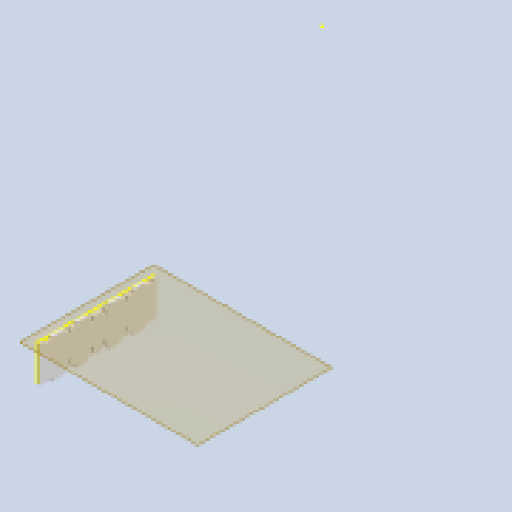
# Autodesk Inventor part: стенка
Saved by Autodesk Inventor 2024.2 (Build 282272000, 272)
## iProperties
Created: 2025-12-09
Part Number: стенка
Material: Типовые
Document SubType Name: Modeling
Designer: katya_notebook
Mass: 65.1748 g
Surface Area: 247.334 cm^2
Volume: 65.1748 cm^3
Density: 1 g/cm^3
Appearance: По умолчанию
Author: katya_notebook
Autodesk Inventor part; units mm, degrees
ref_plane "YZ Plane" through (0, 0, 0) normal (1, 0, 0) x (0, 1, 0)
ref_plane "XZ Plane" through (0, 0, 0) normal (0, 1, 0) x (-1, 0, 0)
ref_plane "РабПлоскость1" through (-475.2675, -216.9886, 379.0883) normal (0, 1, 0) x (-1, 0, 0)
sketch "Эскиз1" plane through (-475.2675, -216.9886, 379.0883) normal (0, 1, 0) x (-1, 0, 0)
  line L0 (135, 97.5) -> (129, 97.5)
  line L1 (129, 97.5) -> (129, -97.5)
  line L2 (129, -97.5) -> (135, -97.5)
  line L3 (135, -97.5) -> (135, 97.5)
  line L4 (135, -97.5) -> (135, 97.5) projected
  line L5 (127, 97.5) -> (62.5237, 97.5) projected
  line L6 (62.5237, -97.5) -> (127, -97.5) projected
  point P0 (-475.2675, -379.0883)
  dimension "d0" = 0
  dimension "d1" = 6
  dimension "d2" = 0
  dimension "d3" = 0
  constraints: 8 end point, 2 parallel, 1 horizontal, 1 perpendicular, 1 vertical alignment
  measures "d0" horizontal extent of L3
  measures "d1" distance of L0.start L0.end
  measures "d2" distance between parallel lines of L6 L2
  measures "d3" distance between parallel lines of L0 L5
ref_plane "РабПлоскость2" through (-610.2675, -276.6936, 277.5883) normal (0, 1, 0) x (0, 0, 1)
extrude "Выдавливание1" add sketch "Эскиз1" against normal up to surface (59.705 mm away)
sketch "Эскиз2" plane through (-610.2675, -216.9886, 281.5883) normal (-1, 0, 0) x (0, 0, 1)
  line L0 (175, -4) -> (187, -4) projected
  line L1 (195, 0) -> (195, -59.705) projected
  line L2 (0, 0) -> (195, 0) projected
  line L3 (0, 0) -> (0, -59.705) projected
  point P0 (-281.5883, 216.9886)
  point P1 (195, -59.705)
  point P2 (0, -59.705)
  constraints: 2 other
sketch "Эскиз3" plane through (-610.2675, -276.6936, 281.5883) normal (-1, 0, 0) x (0, 0, 1)
  line L0 (195, 0) -> (0, 0) projected
  line L1 (175, 0) -> (155, 0)
  line L2 (155, 0) -> (155, -5)
  line L3 (155, -5) -> (175, -5)
  line L4 (175, -5) -> (175, 0)
  line L5 (195, 59.705) -> (195, 0) projected
  line L6 (135, 0) -> (115, 0)
  line L7 (115, 0) -> (115, -5)
  line L8 (115, -5) -> (135, -5)
  line L9 (135, -5) -> (135, 0)
  line L10 (20, 0) -> (40, 0)
  line L11 (40, 0) -> (40, -5)
  line L12 (40, -5) -> (20, -5)
  line L13 (20, -5) -> (20, 0)
  line L14 (60, 0) -> (80, 0)
  line L15 (80, 0) -> (80, -5)
  line L16 (80, -5) -> (60, -5)
  line L17 (60, -5) -> (60, 0)
  line L18 (97.5, 27.8525) -> (226.4185, 27.8525)
  line L19 (195, 55.705) -> (0, 55.705)
  line L20 (175, 55.705) -> (155, 55.705)
  line L21 (155, 55.705) -> (155, 60.705)
  line L22 (155, 60.705) -> (175, 60.705)
  line L23 (175, 60.705) -> (175, 55.705)
  line L24 (135, 55.705) -> (115, 55.705)
  line L25 (115, 55.705) -> (115, 60.705)
  line L26 (115, 60.705) -> (135, 60.705)
  line L27 (135, 60.705) -> (135, 55.705)
  line L28 (20, 55.705) -> (40, 55.705)
  line L29 (40, 55.705) -> (40, 60.705)
  line L30 (40, 60.705) -> (20, 60.705)
  line L31 (20, 60.705) -> (20, 55.705)
  line L32 (60, 55.705) -> (80, 55.705)
  line L33 (80, 55.705) -> (80, 60.705)
  line L34 (80, 60.705) -> (60, 60.705)
  line L35 (60, 60.705) -> (60, 55.705)
  point P0 (-281.5883, 276.6936)
  point P1 (40, 55.705)
  point P2 (80, 55.705)
  point P3 (40, 0)
  point P4 (80, 0)
  point P5 (115, 55.705)
  point P6 (155, 55.705)
  point P7 (115, 0)
  point P8 (155, 0)
  dimension "d8" = 5
  dimension "d9" = 20
  dimension "d10" = 20
  dimension "d11" = 20
  dimension "d12" = 20
  dimension "d13" = 5
  dimension "d14" = 20
  dimension "d15" = 20
  dimension "d16" = 20
  dimension "d17" = 20
  dimension "d43" = 5
  constraints: 68 end point, 17 symmetric about line, 8 parallel, 8 point on line, 5 horizontal, 4 perpendicular
  measures "d8" distance of L3.end L1.start
  measures "d9" distance of L2.end L3.end
  measures "d10" distance of L0.start L1.start
  measures "d11" distance of L7.end L8.end
  measures "d12" distance of L1.end L6.start
  measures "d13" distance of L10.end L11.end
  measures "d14" distance of L11.end L12.end
  measures "d15" distance of L10.start L0.end
  measures "d16" distance of L15.end L16.end
  measures "d17" distance of L14.start L10.end
  measures "d43" distance of L16.end L14.start
extrude "Выдавливание3" add sketch "Эскиз3" against normal blind 6
sketch "Эскиз4" plane through (-610.2675, -276.6936, 281.5883) normal (-1, 0, 0) x (0, 0, 1)
  point P0 (-281.5883, 276.6936)
sketch "Эскиз5" plane through (-610.2675, -276.6936, 281.5883) normal (-1, 0, 0) x (0, 0, 1)
  point P0 (-281.5883, 276.6936)
sketch "Эскиз6" plane through (-610.2675, -276.6936, 281.5883) normal (-1, 0, 0) x (0, 0, 1)
  line L0 (111.125, 1.5) -> (104.625, 1.5)
  line L1 (104.625, 1.5) -> (104.625, 4.5)
  line L2 (104.625, 4.5) -> (111.125, 4.5)
  line L3 (111.125, 4.5) -> (111.125, 1.5)
  line L4 (115, 0) -> (115, -5) projected
  line L5 (90.375, 1.5) -> (83.875, 1.5)
  line L6 (83.875, 1.5) -> (83.875, 4.5)
  line L7 (83.875, 4.5) -> (90.375, 4.5)
  line L8 (90.375, 4.5) -> (90.375, 1.5)
  line L9 (111.125, 3) -> (104.625, 3)
  line L10 (115, 0) -> (80, 0) projected
  line L11 (106.125, 6) -> (109.625, 6)
  line L12 (109.625, 6) -> (109.625, 0)
  line L13 (109.625, 0) -> (106.125, 0)
  line L14 (106.125, 0) -> (106.125, 6)
  line L15 (106.125, 6) -> (109.625, 0) construction
  line L16 (109.625, 6) -> (106.125, 0) construction
  line L17 (90.375, 3) -> (83.875, 3)
  line L18 (87.125, 1.5) -> (87.125, 4.5)
  line L19 (85.375, 6) -> (88.875, 6)
  line L20 (88.875, 6) -> (88.875, 0)
  line L21 (88.875, 0) -> (85.375, 0)
  line L22 (85.375, 0) -> (85.375, 6)
  line L23 (85.375, 6) -> (88.875, 0) construction
  line L24 (88.875, 6) -> (85.375, 0) construction
  line L25 (148.25, 1.5) -> (141.75, 1.5)
  line L26 (141.75, 1.5) -> (141.75, 4.5)
  line L27 (141.75, 4.5) -> (148.25, 4.5)
  line L28 (148.25, 4.5) -> (148.25, 1.5)
  line L29 (148.25, 3) -> (141.75, 3)
  line L30 (143.25, 12) -> (146.75, 12)
  line L31 (146.75, 12) -> (146.75, -6)
  line L32 (146.75, -6) -> (143.25, -6)
  line L33 (143.25, -6) -> (143.25, 12)
  line L34 (143.25, 12) -> (146.75, -6) construction
  line L35 (146.75, 12) -> (143.25, -6) construction
  line L36 (155, 0) -> (155, -5) projected
  line L37 (53.25, 1.5) -> (46.75, 1.5)
  line L38 (46.75, 1.5) -> (46.75, 4.5)
  line L39 (46.75, 4.5) -> (53.25, 4.5)
  line L40 (53.25, 4.5) -> (53.25, 1.5)
  line L41 (53.25, 3) -> (46.75, 3)
  line L42 (48.25, 12) -> (51.75, 12)
  line L43 (51.75, 12) -> (51.75, -6)
  line L44 (51.75, -6) -> (48.25, -6)
  line L45 (48.25, -6) -> (48.25, 12)
  line L46 (48.25, 12) -> (51.75, -6) construction
  line L47 (51.75, 12) -> (48.25, -6) construction
  line L48 (60, 0) -> (60, -5) projected
  line L49 (195, 59.705) -> (195, 0) projected
  line L50 (195, 29.8525) -> (88.875, 29.8525)
  line L51 (111.125, 58.205) -> (104.625, 58.205)
  line L52 (104.625, 58.205) -> (104.625, 55.205)
  line L53 (104.625, 55.205) -> (111.125, 55.205)
  line L54 (111.125, 55.205) -> (111.125, 58.205)
  line L55 (115, 59.705) -> (115, 64.705)
  line L56 (90.375, 58.205) -> (83.875, 58.205)
  line L57 (83.875, 58.205) -> (83.875, 55.205)
  line L58 (83.875, 55.205) -> (90.375, 55.205)
  line L59 (90.375, 55.205) -> (90.375, 58.205)
  line L60 (111.125, 56.705) -> (104.625, 56.705)
  line L61 (115, 59.705) -> (80, 59.705)
  line L62 (106.125, 53.705) -> (109.625, 53.705)
  line L63 (109.625, 53.705) -> (109.625, 59.705)
  line L64 (109.625, 59.705) -> (106.125, 59.705)
  line L65 (106.125, 59.705) -> (106.125, 53.705)
  line L66 (106.125, 53.705) -> (109.625, 59.705) construction
  line L67 (109.625, 53.705) -> (106.125, 59.705) construction
  line L68 (90.375, 56.705) -> (83.875, 56.705)
  line L69 (87.125, 58.205) -> (87.125, 55.205)
  line L70 (85.375, 53.705) -> (88.875, 53.705)
  line L71 (88.875, 53.705) -> (88.875, 59.705)
  line L72 (88.875, 59.705) -> (85.375, 59.705)
  line L73 (85.375, 59.705) -> (85.375, 53.705)
  line L74 (85.375, 53.705) -> (88.875, 59.705) construction
  line L75 (88.875, 53.705) -> (85.375, 59.705) construction
  line L76 (146.75, 65.705) -> (143.25, 65.705)
  line L77 (146.75, 47.705) -> (146.75, 65.705)
  line L78 (146.75, 47.705) -> (143.25, 65.705) construction
  line L79 (143.25, 47.705) -> (146.75, 65.705) construction
  line L80 (143.25, 65.705) -> (143.25, 47.705)
  line L81 (141.75, 58.205) -> (141.75, 55.205)
  line L82 (148.25, 58.205) -> (141.75, 58.205)
  line L83 (148.25, 55.205) -> (148.25, 58.205)
  line L84 (141.75, 55.205) -> (148.25, 55.205)
  line L85 (148.25, 56.705) -> (141.75, 56.705)
  line L86 (143.25, 47.705) -> (146.75, 47.705)
  line L87 (155, 59.705) -> (155, 64.705)
  line L88 (51.75, 65.705) -> (48.25, 65.705)
  line L89 (51.75, 47.705) -> (51.75, 65.705)
  line L90 (51.75, 47.705) -> (48.25, 65.705) construction
  line L91 (48.25, 47.705) -> (51.75, 65.705) construction
  line L92 (48.25, 65.705) -> (48.25, 47.705)
  line L93 (46.75, 58.205) -> (46.75, 55.205)
  line L94 (53.25, 58.205) -> (46.75, 58.205)
  line L95 (53.25, 55.205) -> (53.25, 58.205)
  line L96 (46.75, 55.205) -> (53.25, 55.205)
  line L97 (53.25, 56.705) -> (46.75, 56.705)
  line L98 (48.25, 47.705) -> (51.75, 47.705)
  line L99 (60, 59.705) -> (60, 64.705)
  line L100 (109.625, 6) -> (106.125, 6)
  line L101 (106.125, 6) -> (106.125, 12)
  line L102 (106.125, 12) -> (109.625, 12)
  line L103 (109.625, 12) -> (109.625, 6)
  line L104 (88.875, 6) -> (85.375, 6)
  line L105 (85.375, 6) -> (85.375, 12)
  line L106 (85.375, 12) -> (88.875, 12)
  line L107 (88.875, 12) -> (88.875, 6)
  line L108 (109.625, 53.705) -> (106.125, 53.705)
  line L109 (106.125, 53.705) -> (106.125, 47.705)
  line L110 (106.125, 47.705) -> (109.625, 47.705)
  line L111 (109.625, 47.705) -> (109.625, 53.705)
  line L112 (88.875, 53.705) -> (85.375, 53.705)
  line L113 (85.375, 53.705) -> (85.375, 47.705)
  line L114 (85.375, 47.705) -> (88.875, 47.705)
  line L115 (88.875, 47.705) -> (88.875, 53.705)
  point P0 (-281.5883, 276.6936)
  point P1 (115, -2.5)
  point P2 (107.875, 11.6549)
  point P3 (107.875, 3)
  point P4 (99.25, 0)
  point P5 (87.125, 3)
  point P6 (149.0518, 14.6563)
  point P7 (145, 3)
  point P8 (155, -2.5)
  point P9 (49.2049, 25.9501)
  point P10 (50, 3)
  point P11 (60, -2.5)
  point P12 (48.25, 4.5)
  point P13 (48.25, 1.5)
  point P14 (51.75, 1.5)
  point P15 (51.75, 4.5)
  point P16 (88.875, 4.5)
  point P17 (85.375, 4.5)
  point P18 (85.375, 1.5)
  point P19 (85.375, 0)
  point P20 (88.875, 1.5)
  point P21 (106.125, 1.5)
  point P22 (106.125, 0)
  point P23 (109.625, 1.5)
  point P24 (109.625, 4.5)
  point P25 (106.125, 4.5)
  point P26 (143.25, 1.5)
  point P27 (146.75, 1.5)
  point P28 (146.75, 4.5)
  point P29 (143.25, 4.5)
  point P30 (195, 55.705)
  point P31 (115, 62.205)
  point P32 (107.875, 48.0501)
  point P33 (107.875, 56.705)
  point P34 (99.25, 59.705)
  point P35 (87.125, 56.705)
  point P36 (145, 56.705)
  point P37 (149.0518, 45.0486)
  point P38 (155, 62.205)
  point P39 (50, 56.705)
  point P40 (60, 62.205)
  point P41 (51.75, 55.205)
  point P42 (51.75, 58.205)
  point P43 (48.25, 58.205)
  point P44 (48.25, 55.205)
  point P45 (88.875, 55.205)
  point P46 (88.875, 58.205)
  point P47 (85.375, 55.705)
  point P48 (85.375, 58.205)
  point P49 (85.375, 55.205)
  point P50 (106.125, 58.205)
  point P51 (106.125, 55.205)
  point P52 (109.625, 55.205)
  point P53 (109.625, 58.205)
  point P54 (143.25, 58.205)
  point P55 (143.25, 55.205)
  point P56 (146.75, 55.205)
  point P57 (146.75, 58.205)
  point P58 (85.375, 59.705)
  point P59 (85.375, 53.705)
  point P60 (106.125, 53.705)
  point P61 (85.375, 6)
  point P62 (106.125, 6)
  point P63 (85.375, 0)
  point P64 (85.375, 59.705)
  point P65 (85.375, 53.705)
  point P66 (85.375, 6)
  dimension "d0" = 0
  dimension "d20" = 6.5
  dimension "d21" = 3
  dimension "d22" = 3.875
  dimension "d26" = 6.5
  dimension "d27" = 3
  dimension "d29" = 3
  dimension "d30" = 3.5
  dimension "d32" = 3.5
  dimension "d33" = 6.5
  dimension "d34" = 3
  dimension "d35" = 3.5
  dimension "d36" = 8.25
  dimension "d37" = 6.5
  dimension "d38" = 3
  dimension "d39" = 3.5
  dimension "d40" = 8.25
  dimension "d46" = 6
  dimension "d47" = 6
  constraints: 222 end point, 59 symmetric about line, 26 midpoint, 24 parallel, 13 horizontal, 13 perpendicular, 6 point on line, 5 collinear
  measures "d20" distance of L0.start L0.end
  measures "d21" distance of L0.end L1.end
  measures "d22" horizontal distance of L9.start point (115, -2.5)
  measures "d26" distance of L5.start L5.end
  measures "d27" distance of L5.end L6.end
  measures "d29" distance from line of L10 point (107.875, 3)
  measures "d30" distance of L12.end L13.end
  measures "d32" distance of L21.end L20.end
  measures "d33" distance of L25.start L26.start
  measures "d34" distance of L26.start L26.end
  measures "d35" distance of L32.start L32.end
  measures "d36" distance from line of L31 point (155, -2.5)
  measures "d37" distance of L37.start L38.start
  measures "d38" distance of L38.start L38.end
  measures "d39" distance of L44.start L44.end
  measures "d40" distance from line of L43 point (60, -2.5)
  measures "d46" distance of L100.end L101.end
  measures "d47" distance of L108.end L109.end
extrude "Выдавливание4" cut sketch "Эскиз6" against normal blind 6
sketch "Эскиз7" plane through (-610.2675, -276.6936, 281.5883) normal (-1, 0, 0) x (0, 0, 1)
  line L0 (175, 55.705) -> (187, 55.705) projected
  line L1 (195, 59.705) -> (195, 0) projected
  line L2 (175, 59.705) -> (195, 59.705) projected
  line L3 (175, 59.705) -> (175, 55.705) projected
  line L4 (155, 55.705) -> (155, 59.705) projected
  line L5 (135, 55.705) -> (155, 55.705) projected
  line L6 (135, 59.705) -> (135, 55.705) projected
  line L7 (135, 59.705) -> (155, 59.705) projected
  line L8 (80, 55.705) -> (115, 55.705) projected
  line L9 (115, 55.705) -> (115, 59.705) projected
  line L10 (80, 59.705) -> (80, 55.705) projected
  line L11 (80, 59.705) -> (115, 59.705) projected
  line L12 (60, 55.705) -> (60, 59.705) projected
  line L13 (40, 55.705) -> (60, 55.705) projected
  line L14 (40, 59.705) -> (60, 59.705) projected
  line L15 (40, 59.705) -> (40, 55.705) projected
  line L16 (175, 55.705) -> (187, 55.705) projected
  line L17 (0, 59.705) -> (20, 59.705) projected
  line L18 (0, 59.705) -> (0, 0) projected
  point P0 (-281.5883, 276.6936)
  point P1 (195, 0)
  point P2 (0, 0)
  point P3 (175, 59.705)
  constraints: 2 other
extrude "Выдавливание5" cut sketch "Эскиз7" against normal blind 6
sketch "Эскиз8" plane through (-610.2675, -276.6936, 281.5883) normal (-1, 0, 0) x (0, 0, 1)
  line L0 (187, 59.705) -> (187, 55.705) projected
  line L1 (175, 59.705) -> (175, 55.705) projected
  line L2 (187, 55.705) -> (175, 55.705)
  line L3 (175, 55.705) -> (175, 59.705)
  line L4 (175, 59.705) -> (187, 59.705)
  line L5 (187, 59.705) -> (187, 55.705)
  line L6 (20, 55.705) -> (20, 59.705) projected
  line L7 (8, 55.705) -> (8, 59.705) projected
  line L8 (20, 55.705) -> (8, 55.705)
  line L9 (8, 55.705) -> (8, 59.705)
  line L10 (8, 59.705) -> (20, 59.705)
  line L11 (20, 59.705) -> (20, 55.705)
  point P0 (-281.5883, 276.6936)
  point P1 (8, 55.705)
  point P2 (20, 59.705)
  point P3 (175, 55.705)
  point P4 (187, 59.705)
  constraints: 16 end point, 4 parallel, 2 horizontal, 2 perpendicular
extrude "Выдавливание6" cut sketch "Эскиз8" against normal blind 10
sketch "Эскиз9" plane through (-610.2675, -276.6936, 281.5883) normal (-1, 0, 0) x (0, 0, 1)
  line L0 (163.4276, 22.0483) -> (4.2698, 22.0483) construction
  line L1 (4.2698, 22.0483) -> (4.2698, 35.3902) construction
  line L2 (4.2698, 35.3902) -> (163.4276, 35.3902) construction
  line L3 (163.4276, 35.3902) -> (163.4276, 22.0483) construction
  spline S0 degree 2 poles (156.433, 31.3837) (156.433, 32.4939) (157.9966, 34.0483) (159.1069, 34.0483) knots 0 0 0 1 2 2 2
  line L4 (159.1069, 34.0483) -> (159.9303, 34.0483)
  spline S1 degree 2 poles (159.9303, 34.0483) (161.0406, 34.0483) (162.5949, 32.4939) (162.5949, 31.3837) knots 0 0 0 1 2 2 2
  line L5 (162.5949, 31.3837) -> (162.5949, 24.7499)
  spline S2 degree 2 poles (162.5949, 24.7499) (162.5949, 23.6489) (161.0406, 22.0945) (159.9303, 22.0945) knots 0 0 0 1 2 2 2
  line L6 (159.9303, 22.0945) -> (159.1069, 22.0945)
  spline S3 degree 2 poles (159.1069, 22.0945) (157.9966, 22.0945) (156.433, 23.6489) (156.433, 24.7499) knots 0 0 0 1 2 2 2
  line L7 (156.433, 24.7499) -> (156.433, 31.3837)
  line L8 (157.6173, 31.3837) -> (157.6173, 24.7499)
  spline S4 degree 2 poles (157.6173, 24.7499) (157.6173, 24.1393) (158.4962, 23.2696) (159.1069, 23.2696) knots 0 0 0 1 2 2 2
  line L9 (159.1069, 23.2696) -> (159.9303, 23.2696)
  spline S5 degree 2 poles (159.9303, 23.2696) (160.5317, 23.2696) (161.4106, 24.1485) (161.4106, 24.7499) knots 0 0 0 1 2 2 2
  line L10 (161.4106, 24.7499) -> (161.4106, 31.3837)
  spline S6 degree 2 poles (161.4106, 31.3837) (161.4106, 31.9943) (160.5317, 32.8733) (159.9303, 32.8733) knots 0 0 0 1 2 2 2
  line L11 (159.9303, 32.8733) -> (159.1069, 32.8733)
  spline S7 degree 2 poles (159.1069, 32.8733) (158.4962, 32.8733) (157.6173, 32.0036) (157.6173, 31.3837) knots 0 0 0 1 2 2 2
  spline S8 degree 2 poles (149.6419, 33.4561) (149.6419, 34.0483) (150.2341, 34.0483) knots 0 0 0 1 1 1
  spline S9 degree 2 poles (150.2341, 34.0483) (150.8262, 34.0483) (150.8262, 33.4561) knots 0 0 0 1 1 1
  line L12 (150.8262, 33.4561) -> (150.8262, 26.5911)
  line L13 (150.8262, 26.5911) -> (152.251, 26.5911)
  line L14 (152.251, 26.5911) -> (153.8239, 33.6504)
  spline S10 degree 2 poles (153.8239, 33.6504) (153.9164, 34.0483) (154.379, 34.0483) knots 0 0 0 1 1 1
  spline S11 degree 2 poles (154.379, 34.0483) (154.9712, 34.0483) (154.9712, 33.4746) knots 0 0 0 1 1 1
  spline S12 degree 2 poles (154.9712, 33.4746) (154.9712, 33.4006) (154.9619, 33.3451) knots 0 0 0 1 1 1
  line L15 (154.9619, 33.3451) -> (153.2873, 25.8046)
  spline S13 degree 2 poles (153.2873, 25.8046) (153.1948, 25.416) (152.7229, 25.416) knots 0 0 0 1 1 1
  line L16 (152.7229, 25.416) -> (150.2341, 25.416)
  spline S14 degree 2 poles (150.2341, 25.416) (149.6419, 25.416) (149.6419, 25.9989) knots 0 0 0 1 1 1
  line L17 (149.6419, 25.9989) -> (149.6419, 33.4561)
  spline S15 degree 2 poles (142.8694, 33.4561) (142.8694, 34.0483) (143.4615, 34.0483) knots 0 0 0 1 1 1
  line L18 (143.4615, 34.0483) -> (146.3574, 34.0483)
  spline S16 degree 2 poles (146.3574, 34.0483) (147.1254, 34.0483) (148.1894, 32.975) (148.1894, 32.2164) knots 0 0 0 1 2 2 2
  line L19 (148.1894, 32.2164) -> (148.1894, 25.9989)
  spline S17 degree 2 poles (148.1894, 25.9989) (148.1894, 25.416) (147.5972, 25.416) knots 0 0 0 1 1 1
  spline S18 degree 2 poles (147.5972, 25.416) (147.0051, 25.416) (147.0051, 25.9989) knots 0 0 0 1 1 1
  line L20 (147.0051, 25.9989) -> (147.0051, 32.2071)
  spline S19 degree 2 poles (147.0051, 32.2071) (147.0051, 32.4847) (146.6165, 32.8733) (146.3574, 32.8733) knots 0 0 0 1 2 2 2
  line L21 (146.3574, 32.8733) -> (144.0537, 32.8733)
  line L22 (144.0537, 32.8733) -> (144.0537, 25.9989)
  spline S20 degree 2 poles (144.0537, 25.9989) (144.0537, 25.416) (143.4615, 25.416) knots 0 0 0 1 1 1
  spline S21 degree 2 poles (143.4615, 25.416) (142.8694, 25.416) (142.8694, 25.9989) knots 0 0 0 1 1 1
  line L23 (142.8694, 25.9989) -> (142.8694, 33.4561)
  spline S22 degree 2 poles (136.0783, 32.2164) (136.0783, 32.9658) (137.1516, 34.0483) (137.9288, 34.0483) knots 0 0 0 1 2 2 2
  line L24 (137.9288, 34.0483) -> (139.5664, 34.0483)
  spline S23 degree 2 poles (139.5664, 34.0483) (140.3436, 34.0483) (141.4168, 32.975) (141.4168, 32.2164) knots 0 0 0 1 2 2 2
  line L25 (141.4168, 32.2164) -> (141.4168, 23.9172)
  spline S24 degree 2 poles (141.4168, 23.9172) (141.4168, 23.066) (140.8432, 22.5664) knots 0 0 0 1 1 1
  spline S25 degree 2 poles (140.8432, 22.5664) (140.3343, 22.1038) (139.5849, 22.1038) knots 0 0 0 1 1 1
  spline S26 degree 2 poles (139.5849, 22.1038) (138.8447, 22.1038) (138.3266, 22.5664) knots 0 0 0 1 1 1
  spline S27 degree 2 poles (138.3266, 22.5664) (137.753, 23.0753) (137.753, 23.9265) knots 0 0 0 1 1 1
  spline S28 degree 2 poles (137.753, 23.9265) (137.753, 24.5741) (138.1786, 25.083) knots 0 0 0 1 1 1
  spline S29 degree 2 poles (138.1786, 25.083) (138.5301, 25.3698) (138.8817, 25.416) knots 0 0 0 1 1 1
  line L26 (138.8817, 25.416) -> (137.9288, 25.416)
  spline S30 degree 2 poles (137.9288, 25.416) (137.1516, 25.416) (136.0783, 26.4893) (136.0783, 27.2387) knots 0 0 0 1 2 2 2
  line L27 (136.0783, 27.2387) -> (136.0783, 32.2164)
  line L28 (137.2626, 32.2071) -> (137.2626, 27.2387)
  spline S31 degree 2 poles (137.2626, 27.2387) (137.2626, 26.9797) (137.6512, 26.5911) (137.9288, 26.5911) knots 0 0 0 1 2 2 2
  line L29 (137.9288, 26.5911) -> (139.5664, 26.5911)
  spline S32 degree 2 poles (139.5664, 26.5911) (139.8439, 26.5911) (140.2325, 26.9797) (140.2325, 27.2387) knots 0 0 0 1 2 2 2
  line L30 (140.2325, 27.2387) -> (140.2325, 32.2071)
  spline S33 degree 2 poles (140.2325, 32.2071) (140.2325, 32.4847) (139.8439, 32.8733) (139.5664, 32.8733) knots 0 0 0 1 2 2 2
  line L31 (139.5664, 32.8733) -> (137.9288, 32.8733)
  spline S34 degree 2 poles (137.9288, 32.8733) (137.6512, 32.8733) (137.2626, 32.4847) (137.2626, 32.2071) knots 0 0 0 1 2 2 2
  spline S35 degree 2 poles (138.928, 23.9265) (138.928, 23.6119) (139.3073, 23.2696) (139.5756, 23.2696) knots 0 0 0 1 2 2 2
  spline S36 degree 2 poles (139.5756, 23.2696) (139.8532, 23.2696) (140.1585, 23.4731) knots 0 0 0 1 1 1
  spline S37 degree 2 poles (140.1585, 23.4731) (140.2325, 23.6119) (140.2325, 23.9265) knots 0 0 0 1 1 1
  line L32 (140.2325, 23.9265) -> (140.2325, 25.4068)
  spline S38 degree 2 poles (140.2325, 25.4068) (139.6774, 24.9164) (139.187, 24.4168) knots 0 0 0 1 1 1
  spline S39 degree 2 poles (139.187, 24.4168) (138.928, 24.167) (138.928, 23.9265) knots 0 0 0 1 1 1
  spline S40 degree 2 poles (129.278, 26.0267) (129.278, 26.2395) (129.4353, 26.4153) knots 0 0 0 1 1 1
  spline S41 degree 2 poles (129.4353, 26.4153) (130.7306, 27.8401) (131.9611, 29.1446) knots 0 0 0 1 1 1
  line L33 (131.9611, 29.1446) -> (129.3891, 33.1508)
  spline S42 degree 2 poles (129.3891, 33.1508) (129.2965, 33.2989) (129.2965, 33.4561) knots 0 0 0 1 1 1
  spline S43 degree 2 poles (129.2965, 33.4561) (129.2965, 33.7059) (129.6666, 34.0483) (129.8979, 34.0483) knots 0 0 0 1 2 2 2
  spline S44 degree 2 poles (129.8979, 34.0483) (130.2032, 34.0483) (130.4068, 33.6412) knots 0 0 0 1 1 1
  line L34 (130.4068, 33.6412) -> (132.7383, 29.9403)
  spline S45 degree 2 poles (132.7383, 29.9403) (132.8123, 30.1439) (133.4415, 30.8378) knots 0 0 0 1 1 1
  line L35 (133.4415, 30.8378) -> (133.4415, 33.4561)
  spline S46 degree 2 poles (133.4415, 33.4561) (133.4415, 34.0483) (134.0336, 34.0483) knots 0 0 0 1 1 1
  spline S47 degree 2 poles (134.0336, 34.0483) (134.6258, 34.0483) (134.6258, 33.4561) knots 0 0 0 1 1 1
  line L36 (134.6258, 33.4561) -> (134.6258, 25.9989)
  spline S48 degree 2 poles (134.6258, 25.9989) (134.6258, 25.416) (134.0336, 25.416) knots 0 0 0 1 1 1
  spline S49 degree 2 poles (134.0336, 25.416) (133.4415, 25.416) (133.4415, 25.9989) knots 0 0 0 1 1 1
  line L37 (133.4415, 25.9989) -> (133.4415, 29.3482)
  line L38 (133.4415, 29.3482) -> (130.3605, 25.7121)
  spline S50 degree 2 poles (130.3605, 25.7121) (130.1292, 25.4345) (129.8887, 25.4345) knots 0 0 0 1 1 1
  spline S51 degree 2 poles (129.8887, 25.4345) (129.6389, 25.4345) (129.278, 25.7954) (129.278, 26.0267) knots 0 0 0 1 2 2 2
  spline S52 degree 2 poles (122.524, 32.2164) (122.524, 32.975) (123.5972, 34.0483) (124.3559, 34.0483) knots 0 0 0 1 2 2 2
  line L39 (124.3559, 34.0483) -> (126.012, 34.0483)
  spline S53 degree 2 poles (126.012, 34.0483) (126.78, 34.0483) (127.8439, 32.975) (127.8439, 32.2164) knots 0 0 0 1 2 2 2
  line L40 (127.8439, 32.2164) -> (127.8439, 27.2387)
  spline S54 degree 2 poles (127.8439, 27.2387) (127.8439, 26.4893) (126.7707, 25.416) (126.012, 25.416) knots 0 0 0 1 2 2 2
  line L41 (126.012, 25.416) -> (124.3559, 25.416)
  spline S55 degree 2 poles (124.3559, 25.416) (123.6065, 25.416) (122.524, 26.4985) (122.524, 27.2387) knots 0 0 0 1 2 2 2
  line L42 (122.524, 27.2387) -> (122.524, 32.2164)
  line L43 (123.7083, 32.2071) -> (123.7083, 27.2387)
  spline S56 degree 2 poles (123.7083, 27.2387) (123.7083, 26.9797) (124.0968, 26.5911) (124.3559, 26.5911) knots 0 0 0 1 2 2 2
  line L44 (124.3559, 26.5911) -> (126.012, 26.5911)
  spline S57 degree 2 poles (126.012, 26.5911) (126.2711, 26.5911) (126.6597, 26.9797) (126.6597, 27.2387) knots 0 0 0 1 2 2 2
  line L45 (126.6597, 27.2387) -> (126.6597, 32.2071)
  spline S58 degree 2 poles (126.6597, 32.2071) (126.6597, 32.4847) (126.2711, 32.8733) (126.012, 32.8733) knots 0 0 0 1 2 2 2
  line L46 (126.012, 32.8733) -> (124.3559, 32.8733)
  spline S59 degree 2 poles (124.3559, 32.8733) (124.0968, 32.8733) (123.7083, 32.4847) (123.7083, 32.2071) knots 0 0 0 1 2 2 2
  spline S60 degree 2 poles (115.7329, 32.2164) (115.7329, 32.9658) (116.8062, 34.0483) (117.5833, 34.0483) knots 0 0 0 1 2 2 2
  line L47 (117.5833, 34.0483) -> (119.221, 34.0483)
  spline S61 degree 2 poles (119.221, 34.0483) (119.9982, 34.0483) (121.0714, 32.975) (121.0714, 32.2164) knots 0 0 0 1 2 2 2
  line L48 (121.0714, 32.2164) -> (121.0714, 23.9172)
  spline S62 degree 2 poles (121.0714, 23.9172) (121.0714, 23.066) (120.4978, 22.5664) knots 0 0 0 1 1 1
  spline S63 degree 2 poles (120.4978, 22.5664) (119.9889, 22.1038) (119.2395, 22.1038) knots 0 0 0 1 1 1
  spline S64 degree 2 poles (119.2395, 22.1038) (118.4993, 22.1038) (117.9812, 22.5664) knots 0 0 0 1 1 1
  spline S65 degree 2 poles (117.9812, 22.5664) (117.4076, 23.0753) (117.4076, 23.9265) knots 0 0 0 1 1 1
  spline S66 degree 2 poles (117.4076, 23.9265) (117.4076, 24.5741) (117.8332, 25.083) knots 0 0 0 1 1 1
  spline S67 degree 2 poles (117.8332, 25.083) (118.1847, 25.3698) (118.5363, 25.416) knots 0 0 0 1 1 1
  line L49 (118.5363, 25.416) -> (117.5833, 25.416)
  spline S68 degree 2 poles (117.5833, 25.416) (116.8062, 25.416) (115.7329, 26.4893) (115.7329, 27.2387) knots 0 0 0 1 2 2 2
  line L50 (115.7329, 27.2387) -> (115.7329, 32.2164)
  line L51 (116.9172, 32.2071) -> (116.9172, 27.2387)
  spline S69 degree 2 poles (116.9172, 27.2387) (116.9172, 26.9797) (117.3058, 26.5911) (117.5833, 26.5911) knots 0 0 0 1 2 2 2
  line L52 (117.5833, 26.5911) -> (119.221, 26.5911)
  spline S70 degree 2 poles (119.221, 26.5911) (119.4985, 26.5911) (119.8871, 26.9797) (119.8871, 27.2387) knots 0 0 0 1 2 2 2
  line L53 (119.8871, 27.2387) -> (119.8871, 32.2071)
  spline S71 degree 2 poles (119.8871, 32.2071) (119.8871, 32.4847) (119.4985, 32.8733) (119.221, 32.8733) knots 0 0 0 1 2 2 2
  line L54 (119.221, 32.8733) -> (117.5833, 32.8733)
  spline S72 degree 2 poles (117.5833, 32.8733) (117.3058, 32.8733) (116.9172, 32.4847) (116.9172, 32.2071) knots 0 0 0 1 2 2 2
  spline S73 degree 2 poles (118.5826, 23.9265) (118.5826, 23.6119) (118.9619, 23.2696) (119.2302, 23.2696) knots 0 0 0 1 2 2 2
  spline S74 degree 2 poles (119.2302, 23.2696) (119.5078, 23.2696) (119.8131, 23.4731) knots 0 0 0 1 1 1
  spline S75 degree 2 poles (119.8131, 23.4731) (119.8871, 23.6119) (119.8871, 23.9265) knots 0 0 0 1 1 1
  line L55 (119.8871, 23.9265) -> (119.8871, 25.4068)
  spline S76 degree 2 poles (119.8871, 25.4068) (119.332, 24.9164) (118.8416, 24.4168) knots 0 0 0 1 1 1
  spline S77 degree 2 poles (118.8416, 24.4168) (118.5826, 24.167) (118.5826, 23.9265) knots 0 0 0 1 1 1
  spline S78 degree 2 poles (109.7838, 32.2164) (109.7838, 32.975) (110.8571, 34.0483) (111.625, 34.0483) knots 0 0 0 1 2 2 2
  line L56 (111.625, 34.0483) -> (113.6975, 34.0483)
  spline S79 degree 2 poles (113.6975, 34.0483) (114.2896, 34.0483) (114.2896, 33.4561) knots 0 0 0 1 1 1
  line L57 (114.2896, 33.4561) -> (114.2896, 25.9989)
  spline S80 degree 2 poles (114.2896, 25.9989) (114.2896, 25.416) (113.6975, 25.416) knots 0 0 0 1 1 1
  spline S81 degree 2 poles (113.6975, 25.416) (113.1053, 25.416) (113.1053, 25.9989) knots 0 0 0 1 1 1
  line L58 (113.1053, 25.9989) -> (113.1053, 29.1446)
  line L59 (113.1053, 29.1446) -> (111.6157, 29.1446)
  spline S82 degree 2 poles (111.6157, 29.1446) (110.8571, 29.1446) (109.7838, 30.2271) (109.7838, 30.9673) knots 0 0 0 1 2 2 2
  line L60 (109.7838, 30.9673) -> (109.7838, 32.2164)
  spline S83 degree 2 poles (108.1277, 33.4561) (108.1277, 34.0483) (108.7198, 34.0483) knots 0 0 0 1 1 1
  spline S84 degree 2 poles (108.7198, 34.0483) (109.312, 34.0483) (109.312, 33.4561) knots 0 0 0 1 1 1
  line L61 (109.312, 33.4561) -> (109.312, 25.9989)
  spline S85 degree 2 poles (109.312, 25.9989) (109.312, 25.416) (108.7198, 25.416) knots 0 0 0 1 1 1
  spline S86 degree 2 poles (108.7198, 25.416) (108.1277, 25.416) (108.1277, 25.9989) knots 0 0 0 1 1 1
  line L62 (108.1277, 25.9989) -> (108.1277, 33.4561)
  line L63 (110.9681, 32.2164) -> (110.9681, 30.9673)
  spline S87 degree 2 poles (110.9681, 30.9673) (110.9681, 30.7083) (111.3567, 30.3197) (111.625, 30.3197) knots 0 0 0 1 2 2 2
  line L64 (111.625, 30.3197) -> (113.1053, 30.3197)
  line L65 (113.1053, 30.3197) -> (113.1053, 32.8733)
  line L66 (113.1053, 32.8733) -> (111.625, 32.8733)
  spline S88 degree 2 poles (111.625, 32.8733) (111.3567, 32.8733) (110.9681, 32.4847) (110.9681, 32.2164) knots 0 0 0 1 2 2 2
  spline S89 degree 2 poles (101.3366, 33.4561) (101.3366, 34.0483) (101.9288, 34.0483) knots 0 0 0 1 1 1
  line L67 (101.9288, 34.0483) -> (104.8247, 34.0483)
  spline S90 degree 2 poles (104.8247, 34.0483) (105.5926, 34.0483) (106.6566, 32.975) (106.6566, 32.2071) knots 0 0 0 1 2 2 2
  line L68 (106.6566, 32.2071) -> (106.6566, 25.9897)
  spline S91 degree 2 poles (106.6566, 25.9897) (106.6566, 25.4068) (106.0645, 25.4068) knots 0 0 0 1 1 1
  spline S92 degree 2 poles (106.0645, 25.4068) (105.4723, 25.4068) (105.4723, 25.9897) knots 0 0 0 1 1 1
  line L69 (105.4723, 25.9897) -> (105.4723, 32.2071)
  spline S93 degree 2 poles (105.4723, 32.2071) (105.4723, 32.4847) (105.0837, 32.8733) (104.8247, 32.8733) knots 0 0 0 1 2 2 2
  line L70 (104.8247, 32.8733) -> (102.5209, 32.8733)
  line L71 (102.5209, 32.8733) -> (102.5209, 25.9897)
  spline S94 degree 2 poles (102.5209, 25.9897) (102.5209, 25.4068) (101.9288, 25.4068) knots 0 0 0 1 1 1
  spline S95 degree 2 poles (101.9288, 25.4068) (101.3366, 25.4068) (101.3366, 25.9897) knots 0 0 0 1 1 1
  line L72 (101.3366, 25.9897) -> (101.3366, 33.4561)
  line L73 (103.1778, 23.2696) -> (104.8154, 23.2696)
  spline S96 degree 2 poles (104.8154, 23.2696) (105.4076, 23.2696) (105.4076, 22.6774) knots 0 0 0 1 1 1
  spline S97 degree 2 poles (105.4076, 22.6774) (105.4076, 22.0945) (104.8154, 22.0945) knots 0 0 0 1 1 1
  line L74 (104.8154, 22.0945) -> (103.1778, 22.0945)
  spline S98 degree 2 poles (103.1778, 22.0945) (102.5857, 22.0945) (102.5857, 22.6774) knots 0 0 0 1 1 1
  spline S99 degree 2 poles (102.5857, 22.6774) (102.5857, 23.2696) (103.1778, 23.2696) knots 0 0 0 1 1 1
  spline S100 degree 2 poles (89.4384, 26.0267) (89.4384, 26.2395) (89.5957, 26.4153) knots 0 0 0 1 1 1
  spline S101 degree 2 poles (89.5957, 26.4153) (90.891, 27.8401) (92.1215, 29.1446) knots 0 0 0 1 1 1
  line L75 (92.1215, 29.1446) -> (89.5494, 33.1508)
  spline S102 degree 2 poles (89.5494, 33.1508) (89.4569, 33.2989) (89.4569, 33.4561) knots 0 0 0 1 1 1
  spline S103 degree 2 poles (89.4569, 33.4561) (89.4569, 33.7059) (89.827, 34.0483) (90.0583, 34.0483) knots 0 0 0 1 2 2 2
  spline S104 degree 2 poles (90.0583, 34.0483) (90.3636, 34.0483) (90.5672, 33.6412) knots 0 0 0 1 1 1
  line L76 (90.5672, 33.6412) -> (92.8987, 29.9403)
  spline S105 degree 2 poles (92.8987, 29.9403) (92.9727, 30.1439) (93.6018, 30.8378) knots 0 0 0 1 1 1
  line L77 (93.6018, 30.8378) -> (93.6018, 33.4561)
  spline S106 degree 2 poles (93.6018, 33.4561) (93.6018, 34.0483) (94.194, 34.0483) knots 0 0 0 1 1 1
  spline S107 degree 2 poles (94.194, 34.0483) (94.7861, 34.0483) (94.7861, 33.4561) knots 0 0 0 1 1 1
  line L78 (94.7861, 33.4561) -> (94.7861, 25.9989)
  spline S108 degree 2 poles (94.7861, 25.9989) (94.7861, 25.416) (94.194, 25.416) knots 0 0 0 1 1 1
  spline S109 degree 2 poles (94.194, 25.416) (93.6018, 25.416) (93.6018, 25.9989) knots 0 0 0 1 1 1
  line L79 (93.6018, 25.9989) -> (93.6018, 29.3482)
  line L80 (93.6018, 29.3482) -> (90.5209, 25.7121)
  spline S110 degree 2 poles (90.5209, 25.7121) (90.2896, 25.4345) (90.049, 25.4345) knots 0 0 0 1 1 1
  spline S111 degree 2 poles (90.049, 25.4345) (89.7992, 25.4345) (89.4384, 25.7954) (89.4384, 26.0267) knots 0 0 0 1 2 2 2
  spline S112 degree 2 poles (81.9164, 33.4654) (81.9164, 34.076) (82.4993, 34.076) knots 0 0 0 1 1 1
  spline S113 degree 2 poles (82.4993, 34.076) (82.9342, 34.076) (83.369, 33.4931) knots 0 0 0 1 1 1
  spline S114 degree 2 poles (83.369, 33.4931) (83.7761, 34.0483) (84.6088, 34.0483) knots 0 0 0 1 1 1
  line L81 (84.6088, 34.0483) -> (86.2649, 34.0483)
  spline S115 degree 2 poles (86.2649, 34.0483) (87.0328, 34.0483) (88.0968, 32.975) (88.0968, 32.2164) knots 0 0 0 1 2 2 2
  line L82 (88.0968, 32.2164) -> (88.0968, 27.2387)
  spline S116 degree 2 poles (88.0968, 27.2387) (88.0968, 26.4893) (87.0236, 25.416) (86.2649, 25.416) knots 0 0 0 1 2 2 2
  line L83 (86.2649, 25.416) -> (83.369, 25.416)
  spline S117 degree 2 poles (83.369, 25.416) (82.7769, 25.416) (82.7769, 25.9989) knots 0 0 0 1 1 1
  line L84 (82.7769, 25.9989) -> (82.7769, 32.2349)
  spline S118 degree 2 poles (82.7769, 32.2349) (82.7769, 32.7437) (82.3235, 32.9288) knots 0 0 0 1 1 1
  spline S119 degree 2 poles (82.3235, 32.9288) (81.9164, 33.0861) (81.9164, 33.4654) knots 0 0 0 1 1 1
  line L85 (83.9611, 32.2071) -> (83.9611, 26.5911)
  line L86 (83.9611, 26.5911) -> (86.2649, 26.5911)
  spline S120 degree 2 poles (86.2649, 26.5911) (86.524, 26.5911) (86.9126, 26.9797) (86.9126, 27.2387) knots 0 0 0 1 2 2 2
  line L87 (86.9126, 27.2387) -> (86.9126, 32.2071)
  spline S121 degree 2 poles (86.9126, 32.2071) (86.9126, 32.4847) (86.524, 32.8733) (86.2649, 32.8733) knots 0 0 0 1 2 2 2
  line L88 (86.2649, 32.8733) -> (84.6088, 32.8733)
  spline S122 degree 2 poles (84.6088, 32.8733) (84.3497, 32.8733) (83.9611, 32.4847) (83.9611, 32.2071) knots 0 0 0 1 2 2 2
  spline S123 degree 2 poles (75.9025, 32.2164) (75.9025, 32.9658) (76.9758, 34.0483) (77.7437, 34.0483) knots 0 0 0 1 2 2 2
  line L89 (77.7437, 34.0483) -> (79.3813, 34.0483)
  spline S124 degree 2 poles (79.3813, 34.0483) (80.1585, 34.0483) (81.2225, 32.975) (81.2225, 32.2164) knots 0 0 0 1 2 2 2
  line L90 (81.2225, 32.2164) -> (81.2225, 27.2387)
  spline S125 degree 2 poles (81.2225, 27.2387) (81.2225, 26.4893) (80.1585, 25.416) (79.3813, 25.416) knots 0 0 0 1 2 2 2
  line L91 (79.3813, 25.416) -> (78.4284, 25.416)
  line L92 (78.4284, 25.416) -> (80.9172, 23.1493)
  spline S126 degree 2 poles (80.9172, 23.1493) (81.278, 22.881) (81.278, 22.6127) knots 0 0 0 1 1 1
  spline S127 degree 2 poles (81.278, 22.6127) (81.278, 22.0945) (80.6304, 22.0945) knots 0 0 0 1 1 1
  line L93 (80.6304, 22.0945) -> (76.4947, 22.0945)
  spline S128 degree 2 poles (76.4947, 22.0945) (75.9025, 22.0945) (75.9025, 22.6774) knots 0 0 0 1 1 1
  spline S129 degree 2 poles (75.9025, 22.6774) (75.9025, 23.2696) (76.4947, 23.2696) knots 0 0 0 1 1 1
  line L94 (76.4947, 23.2696) -> (79.4369, 23.2696)
  line L95 (79.4369, 23.2696) -> (76.3651, 26.0729)
  spline S130 degree 2 poles (76.3651, 26.0729) (75.9025, 26.4893) (75.9025, 27.2387) knots 0 0 0 1 1 1
  line L96 (75.9025, 27.2387) -> (75.9025, 32.2164)
  line L97 (77.0868, 32.2071) -> (77.0868, 27.2387)
  spline S131 degree 2 poles (77.0868, 27.2387) (77.0868, 26.9797) (77.4754, 26.5911) (77.7437, 26.5911) knots 0 0 0 1 2 2 2
  line L98 (77.7437, 26.5911) -> (79.3813, 26.5911)
  spline S132 degree 2 poles (79.3813, 26.5911) (79.6497, 26.5911) (80.0382, 26.9797) (80.0382, 27.2387) knots 0 0 0 1 2 2 2
  line L99 (80.0382, 27.2387) -> (80.0382, 32.2071)
  spline S133 degree 2 poles (80.0382, 32.2071) (80.0382, 32.4847) (79.6497, 32.8733) (79.3813, 32.8733) knots 0 0 0 1 2 2 2
  line L100 (79.3813, 32.8733) -> (77.7437, 32.8733)
  spline S134 degree 2 poles (77.7437, 32.8733) (77.4754, 32.8733) (77.0868, 32.4847) (77.0868, 32.2071) knots 0 0 0 1 2 2 2
  line L101 (73.2564, 34.0575) -> (73.2564, 36.7776)
  spline S135 degree 2 poles (73.2564, 36.7776) (73.2564, 37.3698) (73.8486, 37.3698) knots 0 0 0 1 1 1
  spline S136 degree 2 poles (73.8486, 37.3698) (74.4407, 37.3698) (74.4407, 36.7776) knots 0 0 0 1 1 1
  line L102 (74.4407, 36.7776) -> (74.4407, 25.9989)
  spline S137 degree 2 poles (74.4407, 25.9989) (74.4407, 25.416) (73.8486, 25.416) knots 0 0 0 1 1 1
  line L103 (73.8486, 25.416) -> (70.9434, 25.416)
  spline S138 degree 2 poles (70.9434, 25.416) (70.194, 25.416) (69.1207, 26.4893) (69.1207, 27.2295) knots 0 0 0 1 2 2 2
  line L104 (69.1207, 27.2295) -> (69.1207, 32.2164)
  spline S139 degree 2 poles (69.1207, 32.2164) (69.1207, 32.9658) (70.194, 34.0575) (70.9434, 34.0575) knots 0 0 0 1 2 2 2
  line L105 (70.9434, 34.0575) -> (73.2564, 34.0575)
  line L106 (73.2564, 32.8825) -> (70.9434, 32.8825)
  spline S140 degree 2 poles (70.9434, 32.8825) (70.6843, 32.8825) (70.305, 32.4847) (70.305, 32.2164) knots 0 0 0 1 2 2 2
  line L107 (70.305, 32.2164) -> (70.305, 27.2387)
  spline S141 degree 2 poles (70.305, 27.2387) (70.305, 26.9797) (70.6936, 26.5911) (70.9434, 26.5911) knots 0 0 0 1 2 2 2
  line L108 (70.9434, 26.5911) -> (73.2564, 26.5911)
  line L109 (73.2564, 26.5911) -> (73.2564, 32.8825)
  spline S142 degree 2 poles (62.3389, 33.4561) (62.3389, 34.0483) (62.9311, 34.0483) knots 0 0 0 1 1 1
  line L110 (62.9311, 34.0483) -> (65.827, 34.0483)
  spline S143 degree 2 poles (65.827, 34.0483) (66.5949, 34.0483) (67.6589, 32.975) (67.6589, 32.2164) knots 0 0 0 1 2 2 2
  line L111 (67.6589, 32.2164) -> (67.6589, 25.9989)
  spline S144 degree 2 poles (67.6589, 25.9989) (67.6589, 25.416) (67.0668, 25.416) knots 0 0 0 1 1 1
  spline S145 degree 2 poles (67.0668, 25.416) (66.4746, 25.416) (66.4746, 25.9989) knots 0 0 0 1 1 1
  line L112 (66.4746, 25.9989) -> (66.4746, 32.2071)
  spline S146 degree 2 poles (66.4746, 32.2071) (66.4746, 32.4847) (66.086, 32.8733) (65.827, 32.8733) knots 0 0 0 1 2 2 2
  line L113 (65.827, 32.8733) -> (63.5232, 32.8733)
  line L114 (63.5232, 32.8733) -> (63.5232, 25.9989)
  spline S147 degree 2 poles (63.5232, 25.9989) (63.5232, 25.416) (62.9311, 25.416) knots 0 0 0 1 1 1
  spline S148 degree 2 poles (62.9311, 25.416) (62.3389, 25.416) (62.3389, 25.9989) knots 0 0 0 1 1 1
  line L115 (62.3389, 25.9989) -> (62.3389, 33.4561)
  spline S149 degree 2 poles (55.5571, 32.2164) (55.5571, 32.975) (56.6304, 34.0483) (57.389, 34.0483) knots 0 0 0 1 2 2 2
  line L116 (57.389, 34.0483) -> (59.0452, 34.0483)
  spline S150 degree 2 poles (59.0452, 34.0483) (59.8131, 34.0483) (60.8771, 32.975) (60.8771, 32.2164) knots 0 0 0 1 2 2 2
  line L117 (60.8771, 32.2164) -> (60.8771, 27.2387)
  spline S151 degree 2 poles (60.8771, 27.2387) (60.8771, 26.4893) (59.8039, 25.416) (59.0452, 25.416) knots 0 0 0 1 2 2 2
  line L118 (59.0452, 25.416) -> (57.389, 25.416)
  spline S152 degree 2 poles (57.389, 25.416) (56.6396, 25.416) (55.5571, 26.4985) (55.5571, 27.2387) knots 0 0 0 1 2 2 2
  line L119 (55.5571, 27.2387) -> (55.5571, 32.2164)
  line L120 (56.7414, 32.2071) -> (56.7414, 27.2387)
  spline S153 degree 2 poles (56.7414, 27.2387) (56.7414, 26.9797) (57.13, 26.5911) (57.389, 26.5911) knots 0 0 0 1 2 2 2
  line L121 (57.389, 26.5911) -> (59.0452, 26.5911)
  spline S154 degree 2 poles (59.0452, 26.5911) (59.3042, 26.5911) (59.6928, 26.9797) (59.6928, 27.2387) knots 0 0 0 1 2 2 2
  line L122 (59.6928, 27.2387) -> (59.6928, 32.2071)
  spline S155 degree 2 poles (59.6928, 32.2071) (59.6928, 32.4847) (59.3042, 32.8733) (59.0452, 32.8733) knots 0 0 0 1 2 2 2
  line L123 (59.0452, 32.8733) -> (57.389, 32.8733)
  spline S156 degree 2 poles (57.389, 32.8733) (57.13, 32.8733) (56.7414, 32.4847) (56.7414, 32.2071) knots 0 0 0 1 2 2 2
  spline S157 degree 2 poles (48.7661, 33.4561) (48.7661, 34.0483) (49.3582, 34.0483) knots 0 0 0 1 1 1
  spline S158 degree 2 poles (49.3582, 34.0483) (49.9503, 34.0483) (49.9503, 33.4561) knots 0 0 0 1 1 1
  line L124 (49.9503, 33.4561) -> (49.9503, 26.5911)
  line L125 (49.9503, 26.5911) -> (51.3752, 26.5911)
  line L126 (51.3752, 26.5911) -> (52.948, 33.6504)
  spline S159 degree 2 poles (52.948, 33.6504) (53.0406, 34.0483) (53.5032, 34.0483) knots 0 0 0 1 1 1
  spline S160 degree 2 poles (53.5032, 34.0483) (54.0953, 34.0483) (54.0953, 33.4746) knots 0 0 0 1 1 1
  spline S161 degree 2 poles (54.0953, 33.4746) (54.0953, 33.4006) (54.086, 33.3451) knots 0 0 0 1 1 1
  line L127 (54.086, 33.3451) -> (52.4114, 25.8046)
  spline S162 degree 2 poles (52.4114, 25.8046) (52.3189, 25.416) (51.847, 25.416) knots 0 0 0 1 1 1
  line L128 (51.847, 25.416) -> (49.3582, 25.416)
  spline S163 degree 2 poles (49.3582, 25.416) (48.7661, 25.416) (48.7661, 25.9989) knots 0 0 0 1 1 1
  line L129 (48.7661, 25.9989) -> (48.7661, 33.4561)
  line L130 (46.1292, 30.3197) -> (46.1292, 32.2164)
  spline S164 degree 2 poles (46.1292, 32.2164) (46.1292, 32.4939) (45.7499, 32.8733) (45.4908, 32.8733) knots 0 0 0 1 2 2 2
  line L131 (45.4908, 32.8733) -> (42.5949, 32.8733)
  spline S165 degree 2 poles (42.5949, 32.8733) (42.0028, 32.8733) (42.0028, 33.4561) knots 0 0 0 1 1 1
  spline S166 degree 2 poles (42.0028, 33.4561) (42.0028, 34.0483) (42.5949, 34.0483) knots 0 0 0 1 1 1
  line L132 (42.5949, 34.0483) -> (45.4908, 34.0483)
  spline S167 degree 2 poles (45.4908, 34.0483) (46.2587, 34.0483) (47.3135, 32.975) (47.3135, 32.2164) knots 0 0 0 1 2 2 2
  line L133 (47.3135, 32.2164) -> (47.3135, 27.2387)
  spline S168 degree 2 poles (47.3135, 27.2387) (47.3135, 26.4985) (46.2495, 25.416) (45.4908, 25.416) knots 0 0 0 1 2 2 2
  line L134 (45.4908, 25.416) -> (43.8254, 25.416)
  spline S169 degree 2 poles (43.8254, 25.416) (43.0668, 25.416) (41.9935, 26.4893) (41.9935, 27.248) knots 0 0 0 1 2 2 2
  line L135 (41.9935, 27.248) -> (41.9935, 29.7275)
  spline S170 degree 2 poles (41.9935, 29.7275) (41.9935, 30.3197) (42.5949, 30.3197) knots 0 0 0 1 1 1
  line L136 (42.5949, 30.3197) -> (46.1292, 30.3197)
  line L137 (46.1292, 29.1539) -> (43.1778, 29.1539)
  line L138 (43.1778, 29.1539) -> (43.1778, 27.248)
  spline S171 degree 2 poles (43.1778, 27.248) (43.1778, 26.9797) (43.5664, 26.5911) (43.8254, 26.5911) knots 0 0 0 1 2 2 2
  line L139 (43.8254, 26.5911) -> (45.4908, 26.5911)
  spline S172 degree 2 poles (45.4908, 26.5911) (45.7499, 26.5911) (46.1292, 26.9797) (46.1292, 27.248) knots 0 0 0 1 2 2 2
  line L140 (46.1292, 27.248) -> (46.1292, 29.1539)
  line L141 (37.2102, 26.5911) -> (39.3474, 26.5911)
  line L142 (39.3474, 26.5911) -> (39.3474, 33.4561)
  spline S173 degree 2 poles (39.3474, 33.4561) (39.3474, 34.0483) (39.9395, 34.0483) knots 0 0 0 1 1 1
  spline S174 degree 2 poles (39.9395, 34.0483) (40.5317, 34.0483) (40.5317, 33.4561) knots 0 0 0 1 1 1
  line L143 (40.5317, 33.4561) -> (40.5317, 25.9989)
  spline S175 degree 2 poles (40.5317, 25.9989) (40.5317, 25.416) (39.9395, 25.416) knots 0 0 0 1 1 1
  line L144 (39.9395, 25.416) -> (34.5456, 25.416)
  spline S176 degree 2 poles (34.5456, 25.416) (33.7869, 25.416) (32.7044, 26.4985) (32.7044, 27.2387) knots 0 0 0 1 2 2 2
  line L145 (32.7044, 27.2387) -> (32.7044, 33.4561)
  spline S177 degree 2 poles (32.7044, 33.4561) (32.7044, 34.0483) (33.2965, 34.0483) knots 0 0 0 1 1 1
  spline S178 degree 2 poles (33.2965, 34.0483) (33.8887, 34.0483) (33.8887, 33.4561) knots 0 0 0 1 1 1
  line L146 (33.8887, 33.4561) -> (33.8887, 27.248)
  spline S179 degree 2 poles (33.8887, 27.248) (33.8887, 26.9797) (34.2773, 26.5911) (34.5456, 26.5911) knots 0 0 0 1 2 2 2
  line L147 (34.5456, 26.5911) -> (36.0259, 26.5911)
  line L148 (36.0259, 26.5911) -> (36.0259, 33.4561)
  spline S180 degree 2 poles (36.0259, 33.4561) (36.0259, 34.0483) (36.618, 34.0483) knots 0 0 0 1 1 1
  spline S181 degree 2 poles (36.618, 34.0483) (37.2102, 34.0483) (37.2102, 33.4561) knots 0 0 0 1 1 1
  line L149 (37.2102, 33.4561) -> (37.2102, 26.5911)
  point P0 (-281.5883, 276.6936)
  constraints: 2 other
extrude "Выдавливание7" cut sketch "Эскиз9" against normal blind 1
